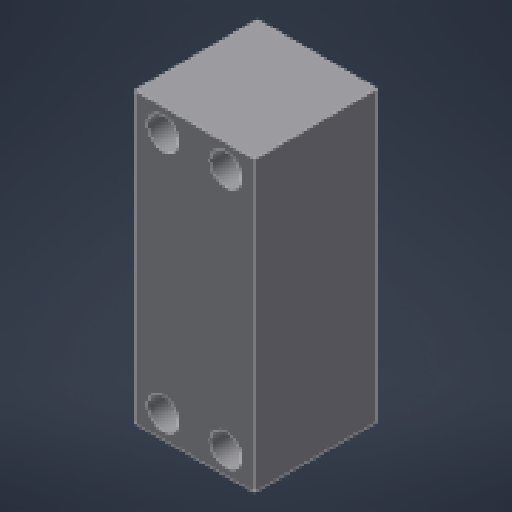
# Autodesk Inventor part: BaseBallScrewSupport
Saved by Autodesk Inventor 2025 (Build 290162000, 162)
## iProperties
Created: 2024-05-17
Part Number: BaseBallScrewSupport
Material: Generic
Document SubType Name: Modeling
Designer: zulet
Density: 1 g/cm^3
Appearance: Default
Author: zulet
Autodesk Inventor part; units mm, degrees
ref_plane "YZ Plane" through (0, 0, 0) normal (1, 0, 0) x (0, 1, 0)
ref_plane "XZ Plane" through (0, 0, 0) normal (0, 1, 0) x (-1, 0, 0)
ref_plane "XY Plane" through (0, 0, 0) normal (0, 0, 1) x (1, 0, 0)
sketch "Sketch1" plane through (0, 0, 0) normal (0, 0, 1) x (1, 0, 0)
  circle A0 centre (10, -42.5) radius 5.5 projected
  circle A1 centre (10, 42.5) radius 5.5 projected
  circle A2 centre (32, -42.5) radius 5.5 projected
  circle A3 centre (32, 42.5) radius 5.5 projected
  line L0 (42, -50.5) -> (42, 50.5) projected
  line L1 (0, 50.5) -> (42, 50.5) projected
  line L2 (0, 50.5) -> (0, -50.5) projected
  line L3 (0, -50.5) -> (42, -50.5) projected
  point P0 (0, 0)
extrude "Extrusion1" add sketch "Sketch1" along normal blind 43
body "Solid1"
